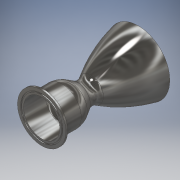
# Autodesk Inventor part: alpha-i
Saved by Autodesk Inventor 2017 (Build 210142000, 142)
## iProperties
Created: 2020-06-16
Part Number: alpha-i
Material: Steel, Mild
Document SubType Name: Modeling
Designer: HAYNIE R&D
Density: 7.85 g/cm^3
Appearance: Semi-Polished
Author: HAYNIE R&D
Autodesk Inventor part; units mm, degrees
ref_plane "YZ Plane" through (0, 0, 0) normal (1, 0, 0) x (0, 1, 0)
ref_plane "XZ Plane" through (0, 0, 0) normal (0, 1, 0) x (-1, 0, 0)
ref_plane "XY Plane" through (0, 0, 0) normal (0, 0, 1) x (1, 0, 0)
sketch "CD Nozzle Sketch" plane through (0, 0, 0) normal (1, 0, 0) x (0, 1, 0)
  line L0 (15.0042, -20) -> (15.0042, -1.5)
  line L1 (15.875, -1.5) -> (15.875, -20)
  arc A0 (6.35, -34.925) -> (15.875, -20) centre (-26.9286, -3.185) ccw
  line L2 (15.875, -1.5) -> (20.0042, -1.5)
  line L3 (20.0042, -1.5) -> (20.0042, 0)
  arc A1 (25.5095, -80) -> (5, -35) centre (-81.2197, -101.4697) ccw
  arc A2 (26.0708, -80) -> (6.35, -34.925) centre (-90.9256, -104.3355) ccw
  arc A3 (5, -35) -> (15.0042, -20) centre (-26.6763, -3.0373) ccw
  line L4 (16.5042, 0) -> (16.5042, -0.75)
  line L5 (16.5042, -0.75) -> (17.5042, -0.75)
  line L6 (17.5042, -0.75) -> (17.5042, 0)
  line L7 (17.5042, 0) -> (20.0042, 0)
  line L8 (0, 1) -> (0, 0)
  line L9 (0, 1) -> (0, 0)
  line L10 (0, 3.175) -> (0, 0)
  line L11 (0, -0.75) -> (0, 0)
  line L12 (26.0708, -80) -> (25.5095, -80)
  line L13 (15.0042, -1.5) -> (15.0042, 0)
  line L14 (15.0042, 0) -> (16.5042, 0)
  line L15 (0, 0) -> (0, -80)
  dimension "d34" = 45
  dimension "d39" = 35
  constraints: 32 end point, 8 point on circle, 6 vertical, 4 centre point, 4 perpendicular, 2 horizontal, 1 collinear
  measures "d34" radius of A3
  measures "d39" vertical distance of A1.end L8.end
revolve "CD Nozzle" add sketch "CD Nozzle Sketch" angle 360 about axis through (0, 0, 0) along (0, 0, -1)
fillet "Fillet14" radius 15 1 edges at (0, -15.875, -20)
fillet "Fillet15" radius 10 1 edges at (0, -6.35, -34.925)
fillet "Fillet16" radius 10 1 edges at (0, -5, -35)
fillet "Fillet17" radius 10 1 edges at (0, -15.0042, -20)
body "Solid2"
